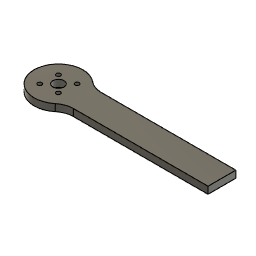
Arm-Test-Coupon (Autodesk Fusion 360 design; units mm, degrees)
Autodesk Fusion 360 part; units mm, degrees
note: some values were not read from the file. Set by a fixed rule: which sketch regions a step uses.
sketch "Sketch1" plane through (0, 0, 0) normal (0, 1, 0) x (1, 0, 0)
  circle A0 centre (0, 0) radius 17.5
  circle A1 centre (0, 0) radius 4
  dimension "d1" = 35
  dimension "d4" = 8
  constraint coincident A0.centre A1.centre
  constraint concentric A0 A1
  measures "d1" diameter of A0
  measures "d4" diameter of A1
extrude "Extrude1" add sketch "Sketch1" along normal blind 5 makes body 1
sketch "Sketch2" plane through (0, 0, 0) normal (0, 1, 0) x (1, 0, 0)
  line L0 (17.5, 10) -> (117.5, 10)
  line L1 (117.5, 10) -> (117.5, -10)
  line L2 (117.5, -10) -> (17.5, -10)
  line L3 (17.5, -10) -> (17.5, 10)
  line L4 (17.5, 10) -> (117.5, -10) construction
  line L5 (117.5, 10) -> (17.5, -10) construction
  circle A0 centre (0, 0) radius 17.5
  point P0 (67.5, 0)
  dimension "d5" = 100
  dimension "d6" = 20
  constraint horizontal L0
  constraint perpendicular L0 L1
  constraint parallel L0 L2
  constraint parallel L1 L3
  constraint coincident L4 P0
  constraint coincident L5 P0
  constraint midpoint L5 P0
  constraint horizontal A0.centre P0
  constraint tangent L3 A0
  measures "d5" distance of L1.end L2.end
  measures "d6" distance of L0 L2
extrude "Extrude2" add sketch "Sketch2" along normal up to surface (5 mm away) separate body contours L0 L1 L2 L3 makes body 2
sketch "Sketch3" plane through (0, 5, 0) normal (0, 1, 0) x (-1, 0, 0)
  circle A0 centre (0, 0) radius 4
  circle A1 centre (0, 0) radius 17.5
  circle A2 centre (0, 0) radius 9.5
  circle A3 centre (0, 0) radius 8
  circle A4 centre (5.6569, -5.6569) radius 1.5
  circle A5 centre (-5.6569, 5.6569) radius 1.5
  circle A6 centre (6.7175, 6.7175) radius 1.5
  circle A7 centre (-6.7175, -6.7175) radius 1.5
  line L0 (0, 0) -> (-6.7175, -6.7175)
  line L1 (0, 0) -> (5.6569, -5.6569)
  line L2 (0, 0) -> (6.7175, 6.7175)
  line L3 (0, 0) -> (-5.6569, 5.6569)
  line L4 (0, 0) -> (-4, 0)
  dimension "d11" = 19
  dimension "d12" = 16
  dimension "d13" = 3
  dimension "d14" = 3
  dimension "d15" = 3
  dimension "d16" = 3
  dimension "d17" = 45
  dimension "d19" = 45
  dimension "d20" = 45
  dimension "d39" = 45
  constraint coincident A0.centre A1.centre
  constraint concentric A2 A3
  constraint coincident A2 A7.centre
  constraint coincident A2 A6.centre
  constraint coincident A3 A4.centre
  constraint coincident A3 A5.centre
  constraint coincident A0 L4.end
  constraint horizontal L4
  constraint coincident A4.centre L1.end
  constraint coincident A6.centre L2.end
  constraint coincident A5.centre L3.end
  constraint coincident A7.centre L0.end
  measures "d11" diameter of A2
  measures "d12" diameter of A3
  measures "d13" diameter of A4
  measures "d14" diameter of A5
  measures "d15" diameter of A6
  measures "d16" diameter of A7
  measures "d17" angle of L0 L4
  measures "d19" angle of L2 L4
  measures "d20" angle of L3 L4
  measures "d39" angle of L1 L4
extrude "Extrude3" cut sketch "Sketch3" against normal blind 5 contours A2 A6 L2 | A2 A6 L2 | A3 A4 L1 | A3 A4 L1 | A3 A5 L3 | A3 A5 L3 | A3 A5 | A2 A6 | A2 A7 L0 | A2 A7 L0 | A3 A4 | A2 A7 bodies 1
sketch "Sketch4" plane through (0, 5, 0) normal (0, 1, 0) x (-1, 0, 0)
  line L0 (-17.5, -10) -> (-17.5, 10)
  line L1 (-17.5, 10) -> (-117.5, 10)
  line L2 (-117.5, 10) -> (-117.5, -10)
  line L3 (-117.5, -10) -> (-17.5, -10)
  arc A0 (-17.5, -10) -> (0, -17.5) centre (-1.8213, 2.4169) ccw
  arc A1 (0, 17.5) -> (-17.5, 10) centre (-1.8213, -2.4169) ccw
  line L4 (0, 17.5) -> (-15, 0)
  line L5 (-15, 0) -> (0, -17.5)
  dimension "d26" = 17.5
  dimension "d28" = 17.5
  dimension "d29" = 20
  dimension "d30" = 20
  constraint coincident L0.start L3.end
  constraint coincident L0.end L1.start
  constraint vertical origin A0.end
  constraint vertical origin A1.start
  measures "d26" distance of origin A0.end
  measures "d28" distance of origin A1.start
  measures "d29" radius of A0
  measures "d30" radius of A1
sketch "Sketch5" plane through (0, 5, 0) normal (0, 1, 0) x (-1, 0, 0)
  line L0 (-17.5, -10) -> (-17.5, 10)
  line L1 (-17.5, 10) -> (-117.5, 10)
  line L2 (-117.5, 10) -> (-117.5, -10)
  line L3 (-117.5, -10) -> (-17.5, -10)
  line L4 (-17.5, -10) -> (-12.5, -10)
  line L5 (-12.5, -10) -> (-12.5, 10)
  line L6 (-12.5, 10) -> (-17.5, 10)
  line L7 (-17.5, 10) -> (-17.5, -10)
  dimension "d33" = 5
  constraint horizontal L4
  constraint vertical L5
  constraint horizontal L6
  constraint vertical L7
  constraint coincident L0.start L3.end
  constraint coincident L0.end L1.start
  measures "d33" distance of L0.start L4.end
extrude "Extrude5" add sketch "Sketch5" against normal blind 5 contours L0 L4 L5 L6 L7 bodies 1 2
fillet "Fillet1" radius 15 2 edges at (14.3614, 2.5, 10) (14.3614, 2.5, -10) on bodies 1
equation "d26 = ( 35 / 2 ) * 1 mm"
